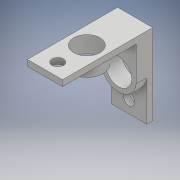
# Autodesk Inventor part: Now as three El L
Saved by Autodesk Inventor 2017 (Build 210142000, 142)
## iProperties
Created: 2017-04-12
Part Number: Now as three El L
Material: Generic
Document SubType Name: Modeling
Designer: andrew
Density: 1 g/cm^3
Appearance: Default
Author: andrew
Autodesk Inventor part; units mm, degrees
ref_plane "YZ Plane" through (0, 0, 0) normal (1, 0, 0) x (0, 1, 0)
ref_plane "XZ Plane" through (0, 0, 0) normal (0, 1, 0) x (-1, 0, 0)
ref_plane "XY Plane" through (0, 0, 0) normal (0, 0, 1) x (1, 0, 0)
sketch "Sketch1" plane through (0, 0, 0) normal (0, 1, 0) x (-1, 0, 0)
  line L0 (-2.2837, -0.9982) -> (0.008, -0.7055) construction
  line L1 (2.6844, -8.3272) -> (2.6844, -12.3272) construction
  line L2 (64.2192, 40.0403) -> (72.5206, 41.3734) construction
  line L3 (64.2192, 39.2192) -> (64.2192, 44.778) construction
  line L4 (-8.9125, -2.5) -> (-8.9125, -6.85) construction
  line L5 (-14.9605, -0.9982) -> (-2.2837, -0.9982) construction
  line L6 (55.95, 41.2553) -> (64.2192, 40.0403) construction
  circle A0 centre (-8.9125, -6.85) radius 4.35
  line L7 (-14.724, -20.8143) -> (-17.8001, -0.7055) construction
  line L8 (-3.0681, -20.8143) -> (0.008, -0.7055) construction
  line L9 (-11.8961, -14.832) -> (-8.8961, -13.1) construction
  line L10 (-8.8961, -13.1) -> (-5.8961, -14.832) construction
  line L11 (-3.0681, -20.8143) -> (-14.724, -20.8143)
  circle A1 centre (-8.8961, -16.5641) radius 1.9
  line L12 (64.2192, 39.2192) -> (64.2192, 43.7357)
  line L13 (-14.9605, -0.9982) -> (-17.8001, -0.7055) construction
  line L14 (-8.8961, -20.8143) -> (-3.0681, -20.8143) construction
  line L15 (-14.724, -20.8143) -> (-3.0681, -20.8143) construction
  line L16 (-8.8258, -6.8795) -> (-8.8093, -6.8795) construction
  line L17 (-5.8961, -14.832) -> (-5.3727, -20.8143) construction
  line L18 (-11.8961, -14.832) -> (-12.4194, -20.8143) construction
  line L19 (-14.2025, 0) -> (-14.2025, -2.5) construction
  line L20 (-14.2025, -2.5) -> (-3.6225, -2.5) construction
  line L21 (-8.9125, -2.5) -> (-8.9125, 0.8916) construction
  line L22 (-3.6225, -20.8143) -> (-14.2025, -20.8143) construction
  line L23 (-3.6225, -20.8143) -> (-14.2025, -20.8143)
  line L24 (-8.9125, -6.85) -> (-13.2625, -6.85) construction
  line L25 (-13.2625, -6.85) -> (-14.2025, -6.85) construction
  line L26 (-3.0681, -20.8143) -> (-3.0681, 0)
  line L27 (-14.724, -20.8143) -> (-14.724, 0) construction
  line L28 (-14.724, 0) -> (-14.2025, 0) construction
  line L29 (-14.724, -20.8143) -> (-14.724, 0)
  line L30 (-14.2025, 0) -> (-14.724, 0)
  line L31 (-3.0681, 0) -> (-3.0681, 4)
  line L32 (-3.0681, 4) -> (-14.724, 4)
  line L33 (-14.724, 0) -> (-14.724, 4)
  point P0 (-0.8016, -0.9982)
  point P1 (-16.9905, -0.9982)
  point P2 (-5.8961, -16.5641)
  point P3 (-8.8961, -16.5641)
  point P4 (-11.8961, -20.8143)
  point P5 (-5.8961, -20.8143)
  dimension "d27" = 3.8
  dimension "d28" = 4
  dimension "d29" = 0.0164
  dimension "d31" = 2.5
  dimension "d36" = 4
  constraints: 68 end point, 9 point on line, 5 vertical, 4 perpendicular, 2 centre point, 2 horizontal, 2 point on circle, 1 collinear, 1 midpoint, 4 other
  measures "d27" diameter of A1
  measures "d28" distance of L1.start L1.end
  measures "d29" distance of L16.start L16.end
  measures "d31" distance of L19.start L19.end
  measures "d36" distance of L26.end L31.end
extrude "Extrusion1" add sketch "Sketch1" along normal blind 2
sketch "Sketch5" plane through (3.0681, 0, 4) normal (0, 0, 1) x (1, 0, 0)
  line L0 (5.6876, -20.2886) -> (8.131, -18.0087) construction
  line L1 (5.8983, -14.0653) -> (5.9147, -14.0653) construction
  line L2 (0, -28) -> (-3.0761, -7.8912) construction
  circle A0 centre (5.8115, -14.0357) radius 4.35
  line L3 (11.6559, -28) -> (14.732, -7.8912) construction
  line L4 (5.8115, -9.6857) -> (5.8115, -14.0357) construction
  line L5 (-22.6444, -7.0488) -> (-20.3527, -6.7561) construction
  circle A1 centre (5.828, -23.7498) radius 1.9
  line L6 (2.828, -22.0178) -> (2.3046, -28) construction
  line L7 (11.6559, -28) -> (0, -28) construction
  line L8 (0, -28) -> (11.6559, -28) construction
  line L9 (5.828, -28) -> (11.6559, -28) construction
  line L10 (8.131, -18.0087) -> (9.3514, -28) construction
  line L11 (2.828, -22.0178) -> (5.6876, -20.2886) construction
  line L12 (-35.3212, -7.0488) -> (-22.6444, -7.0488) construction
  line L13 (-35.3212, -7.0488) -> (-38.1608, -6.7561) construction
  line L14 (0.5215, -7.1857) -> (0.5215, -9.6857) construction
  line L15 (0.5215, -9.6857) -> (11.1015, -9.6857) construction
  line L16 (5.8115, -9.6857) -> (5.8115, -6.2941) construction
  line L17 (11.1015, -28) -> (0.5215, -28) construction
  line L18 (11.1015, -28) -> (0.5215, -28) construction
  line L19 (5.8115, -14.0357) -> (1.4615, -14.0357) construction
  line L20 (1.4615, -14.0357) -> (0.5215, -14.0357) construction
  line L21 (11.6559, -28) -> (11.6559, -7.1857) construction
  line L22 (0, -28) -> (0, -7.1857) construction
  line L23 (-35.0847, -6.0506) -> (-34.5632, -6.0506) construction
  line L24 (0, -28) -> (0, -7.1857) construction
  line L25 (-34.5632, -6.0506) -> (-35.0847, -6.0506) construction
  line L26 (-23.4288, -6.0506) -> (-23.4288, -2.0506) construction
  line L27 (-23.4288, -2.0506) -> (-35.0847, -2.0506) construction
  line L28 (-35.0847, -6.0506) -> (-35.0847, -2.0506) construction
  line L29 (0, 0) -> (11.6559, 0) projected
  line L30 (11.6559, 0) -> (11.6559, 2) projected
  line L31 (0, 2) -> (11.6559, 2) projected
  line L32 (0, 0) -> (0, 2) projected
  line L33 (0, 2) -> (11.6559, 2)
  line L34 (11.6559, 2) -> (11.6559, -28)
  line L35 (11.6559, -28) -> (0, -28)
  line L36 (0, -28) -> (0, 2)
  line L37 (5.828, -28) -> (5.828, -33.9662)
  line L38 (5.828, -28) -> (5.7489, -34.6939)
  point P0 (-4.0686, -7.3836)
  point P1 (8.828, -23.7498)
  point P2 (2.828, -28)
  point P3 (8.828, -28)
  point P4 (-37.3512, -7.0488)
  dimension "d38" = 3.8
  dimension "d40" = 0.0164
  dimension "d41" = 2.5
  dimension "d42" = 4
  dimension "d43" = 30
  constraints: 70 end point, 7 point on line, 6 vertical, 5 perpendicular, 3 equal length, 3 horizontal, 2 centre point, 2 midpoint, 2 point on circle, 4 other
  measures "d38" diameter of A1
  measures "d40" distance of L1.start L1.end
  measures "d41" distance of L14.start L15.start
  measures "d42" distance of L26.start L26.end
  measures "d43" distance of L33.end L34.end
extrude "Extrusion5" add sketch "Sketch5" along normal blind 2
sketch "Sketch6" plane through (3.0681, 0, 4) normal (0, 0, -1) x (-1, 0, 0)
  line L0 (0, 0) -> (-11.6559, 0) projected
  line L1 (-11.6559, -28) -> (-11.6559, 0) projected
  line L2 (0, -28) -> (-11.6559, -28) projected
  line L3 (0, 0) -> (0, -28) projected
  circle A0 centre (-5.828, -23.7498) radius 1.9 projected
  circle A1 centre (-5.8115, -14.0357) radius 4.35 projected
  circle A2 centre (-5.8115, -14.0357) radius 4.35
  circle A3 centre (-5.8115, -14.0357) radius 5.8444
  line L4 (-11.6559, -28) -> (-11.6559, 0) projected
  point P0 (3.0681, 0)
  constraints: 2 centre point, 2 coincident, 1 concentric, 1 tangent
extrude "Extrusion6" add sketch "Sketch6" along normal blind 3.5 contours A3 L3 | L3 A3
chamfer "Chamfer1" distance 0.5 distance2 3.5 1 edges at (14.724, -14.0357, 0.5) measured on face at (3.6321, -14.849, 0.5)
sketch "Sketch8" plane through (0, 0, 0) normal (0, -1, 0) x (1, 0, 0)
  circle A0 centre (8.9125, -6.85) radius 4.35 projected
  circle A1 centre (8.8961, -16.5641) radius 1.9 projected
  line L0 (14.724, -20.8143) -> (3.0681, -20.8143) projected
  line L1 (14.724, 4) -> (14.724, -20.8143) projected
  line L2 (3.0681, 4) -> (14.724, 4) projected
  line L3 (3.0681, -20.8143) -> (3.0681, 4) projected
  arc A2 (3.0681, -6.85) -> (14.724, -7.4691) centre (8.9125, -6.85) ccw
  line L4 (48.394, -18.4641) -> (53.1571, -15.7141)
  line L5 (51.5694, -18.4641) -> (49.9817, -21.2141)
  line L6 (49.9817, -21.2141) -> (46.8063, -21.2141)
  line L7 (46.8063, -21.2141) -> (45.2186, -18.4641)
  line L8 (45.2186, -18.4641) -> (46.8063, -15.7141)
  line L9 (46.8063, -15.7141) -> (49.9817, -15.7141)
  line L10 (49.9817, -15.7141) -> (51.5694, -18.4641)
  line L11 (8.8961, -16.5641) -> (13.6592, -13.8141)
  line L12 (12.0715, -16.5641) -> (10.4838, -19.3141)
  line L13 (10.4838, -19.3141) -> (7.3083, -19.3141)
  line L14 (7.3083, -19.3141) -> (5.7206, -16.5641)
  line L15 (5.7206, -16.5641) -> (7.3083, -13.8141)
  line L16 (7.3083, -13.8141) -> (10.4838, -13.8141)
  line L17 (10.4838, -13.8141) -> (12.0715, -16.5641)
  point P0 (0, 0)
  point P1 (50.7756, -17.0891)
  point P2 (11.2776, -15.1891)
  dimension "d53" = 5.5
  dimension "d54" = 5.5
  constraints: 28 end point, 4 midpoint, 3 coincident, 2 point on circle, 2 point on line, 1 centre point, 1 tangent, 26 other
  measures "d53" distance of L4.start L4.end
  measures "d54" distance of L11.start L11.end
extrude "Extrusion7" add sketch "Sketch8" along normal blind 3.5 contours A2 L3 L2 L1
body "Solid1"
